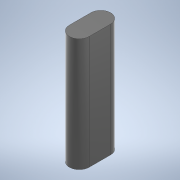
# Autodesk Inventor part: RC_CARS_BATTERY
Saved by Autodesk Inventor 2020 (Build 240168000, 168)
## iProperties
Created: 2019-06-17
Part Number: RC_CARS_BATTERY
Material: 一般
Document SubType Name: Modeling
Designer: shun
Mass: 290 g
Surface Area: 181.188 cm^2
Volume: 130.743 cm^3
Density: 2.2181 g/cm^3
Appearance: 滑らか - 黒
Author: shun
Autodesk Inventor part; units mm, degrees
ref_plane "YZ Plane" through (0, 0, 0) normal (1, 0, 0) x (0, 1, 0)
ref_plane "XZ Plane" through (0, 0, 0) normal (0, 1, 0) x (-1, 0, 0)
ref_plane "XY Plane" through (0, 0, 0) normal (0, 0, 1) x (1, 0, 0)
sketch "スケッチ1" plane through (0, 0, 0) normal (0, 1, 0) x (-1, 0, 0)
  line L0 (11.5, 12.5) -> (-11.5, 12.5) construction
  line L1 (-11.5, 12.5) -> (-11.5, -12.5)
  line L2 (-11.5, -12.5) -> (11.5, -12.5) construction
  line L3 (11.5, -12.5) -> (11.5, 12.5)
  line L4 (11.5, 12.5) -> (-11.5, -12.5) construction
  line L5 (-11.5, 12.5) -> (11.5, -12.5) construction
  line L6 (11.5, 0) -> (-11.5, 0)
  arc A0 (-11.5, -12.5) -> (11.5, -12.5) centre (0, -12.5) ccw
  point P0 (0, 0)
  dimension "d0" = 23
  dimension "d1" = 25
  constraints: 14 end point, 5 midpoint, 2 parallel, 2 point on circle, 1 centre point, 1 horizontal, 1 perpendicular
  measures "d0" distance of L2.end L1.end
  measures "d1" distance of L1.end L0.end
extrude "押し出し1" add sketch "スケッチ1" along normal blind 132
mirror "ミラー1" about plane through (-11.5, 0, 0) normal (0, 0, 1) of "押し出し1"
